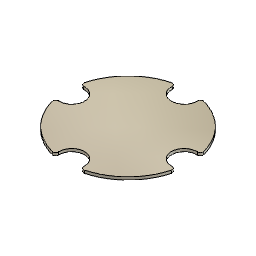
silver contact pieces CAM v3 (Autodesk Fusion 360 archive; units mm, degrees)
design "silver contact part"
Autodesk Fusion 360 part; units mm, degrees
sketch "Sketch1" plane through (0, 0, 0) normal (0, 1, 0) x (1, 0, 0)
  circle A0 centre (0, 0) radius 10 construction
  circle A1 centre (10, 0) radius 2.25
  circle A2 centre (0, 10) radius 2.25
  circle A3 centre (-10, 0) radius 2.25
  circle A4 centre (0, -10) radius 2.25
  circle A5 centre (0, 0) radius 11
  dimension "d1" = 20
  dimension "d2" = 4.5
  dimension "d4" = 360
  dimension "d5" = 22
  constraint coincident A0.centre A5.centre
  constraint coincident A0 A1.centre
  constraint horizontal A0.centre A1.centre
  constraint concentric A0 A5
  measures "d1" diameter of A0
  measures "d2" diameter of A1
  measures "d5" diameter of A5
extrude "Extrude1" add sketch "Sketch1" along normal blind 0.5 contours A1 A2 A3 A4 A5
fillet "Fillet1" radius 0.5 8 edges at (-2.1042, 0.25, 10.7969) (2.1042, 0.25, 10.7969) (-10.7969, 0.25, 2.1042) (-10.7969, 0.25, -2.1042) (-2.1042, 0.25, -10.7969) (2.1042, 0.25, -10.7969) (10.7969, 0.25, -2.1042) (10.7969, 0.25, 2.1042)

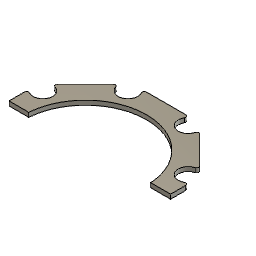
design "stage 1 shield pressure clamp"
Autodesk Fusion 360 part; units mm, degrees
sketch "Sketch1" plane through (0, 0, 0) normal (0, 1, 0) x (1, 0, 0)
  circle A0 centre (0, 0) radius 18 construction
  circle A1 centre (0, 0) radius 14
  circle A2 centre (-16.6298, 6.8883) radius 2.25
  circle A3 centre (-16.6298, -6.8883) radius 2.25
  circle A4 centre (-6.8883, -16.6298) radius 2.25
  circle A5 centre (6.8883, -16.6298) radius 2.25
  circle A6 centre (16.6298, -6.8883) radius 2.25
  circle A7 centre (16.6298, 6.8883) radius 2.25
  circle A8 centre (6.8883, 16.6298) radius 2.25
  circle A9 centre (-6.8883, 16.6298) radius 2.25
  line L0 (-18.5, 7.663) -> (-18.5, -7.663)
  line L1 (-18.5, -7.663) -> (-7.663, -18.5)
  line L2 (-7.663, -18.5) -> (7.663, -18.5)
  line L3 (7.663, -18.5) -> (18.5, -7.663)
  line L4 (18.5, -7.663) -> (18.5, 7.663)
  line L5 (18.5, 7.663) -> (7.663, 18.5)
  line L6 (7.663, 18.5) -> (-7.663, 18.5)
  line L7 (-7.663, 18.5) -> (-18.5, 7.663)
  line L8 (-18.5, 1) -> (18.5, 1)
  point P0 (-16.6298, 6.8883)
  dimension "d1" = 36
  dimension "d2" = 28
  dimension "d3" = 4.5
  dimension "d5" = 360
  dimension "d6" = 18.5
  dimension "d7" = 1
  constraint coincident A0.centre A1.centre
  constraint concentric A0 A1
  constraint coincident A0 P0
  constraint coincident P0 A2.centre
  constraint horizontal A8.centre A9.centre
  constraint horizontal L6
  constraint coincident L0 L8.start
  constraint coincident L4 L8.end
  constraint perpendicular L4 L8
  measures "d1" diameter of A0
  measures "d2" diameter of A1
  measures "d3" diameter of A2
  measures "d6" distance of A0.centre L7
  measures "d7" distance of A0.centre L8
extrude "Extrude1" add sketch "Sketch1" along normal blind 1 contours A1 A2 A7 A8 A9 L0 L4 L5 L6 L7 L8
fillet "Fillet1" radius 0.5 8 edges at (18.5, 0.5, -5.6373) (17.0677, 0.5, -9.0953) (9.0953, 0.5, -17.0677) (5.6373, 0.5, -18.5) (-5.6373, 0.5, -18.5) (-9.0953, 0.5, -17.0677) (-17.0677, 0.5, -9.0953) (-18.5, 0.5, -5.6373)
